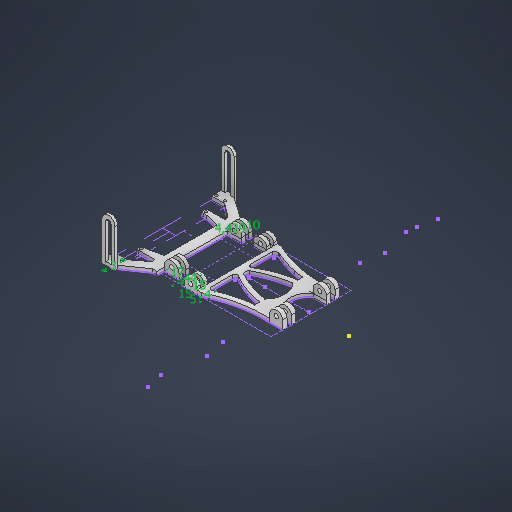
# Autodesk Inventor part: grebla2
Saved by Autodesk Inventor 2026.2 (Build 302298000, 298)
## iProperties
Created: 2026-03-31
Part Number: grebla2
Material: Generic
Document SubType Name: Modeling
Designer: Iosif
Density: 1 g/cm^3
Appearance: Default
Author: Iosif
Autodesk Inventor part; units mm, degrees
ref_plane "YZ Plane" through (0, 0, 0) normal (1, 0, 0) x (0, 1, 0)
ref_plane "XZ Plane" through (0, 0, 0) normal (0, 1, 0) x (-1, 0, 0)
ref_plane "XY Plane" through (0, 0, 0) normal (0, 0, 1) x (1, 0, 0)
sketch "Sketch1" plane through (0, 0, 0) normal (0, 1, 0) x (-1, 0, 0)
  line L0 (197.8218, 40) -> (201.8218, 40)
  arc A0 (201.8218, 34) -> (201.8218, 40) centre (201.8218, 37) ccw
  line L1 (201.8218, 34) -> (197.8218, 34)
  line L2 (197.8218, -34) -> (201.8218, -34)
  arc A1 (201.8218, -40) -> (201.8218, -34) centre (201.8218, -37) ccw
  line L3 (201.8218, -40) -> (197.8218, -40)
  line L4 (214.3218, -64) -> (214.3218, -59)
  line L5 (214.3218, -59) -> (214.3218, -56)
  line L6 (214.3218, -56) -> (199.3218, -56)
  line L7 (199.3218, 56) -> (214.3218, 56)
  line L8 (214.3218, 56) -> (214.3218, 59)
  line L9 (214.3218, 59) -> (214.3218, 64)
  line L10 (197.8218, 34) -> (182.1137, 30.3299)
  line L11 (182.1137, 30.3299) -> (182.1137, -30.3299)
  line L12 (182.1137, -30.3299) -> (197.8218, -34)
  line L13 (199.3218, 56) -> (184.6899, 44.9596)
  arc A2 (184.6899, 44.9596) -> (183.5786, 40) centre (187.0547, 41.8254) ccw
  line L14 (183.5786, 40) -> (197.8218, 40)
  line L15 (197.8218, -40) -> (183.5786, -40)
  arc A3 (183.5786, -40) -> (184.6899, -44.9596) centre (187.0547, -41.8254) ccw
  line L16 (184.6899, -44.9596) -> (199.3218, -56)
  line L17 (170.1376, 0) -> (214.3218, 0)
  line L18 (214.3218, 0) -> (214.3218, -64)
  line L19 (214.3218, 0) -> (214.3218, 64)
  line L20 (206.8218, 0) -> (206.8218, 59)
  line L21 (206.8218, 59) -> (214.3218, 59)
  line L22 (206.8218, 57.5) -> (211.8218, 57.5)
  line L23 (211.8218, 57.5) -> (211.8218, 59)
  line L24 (206.8218, 57.5) -> (201.8218, 57.5)
  line L25 (201.8218, 57.5) -> (201.8218, 59)
  circle A4 centre (211.8218, 59) radius 1.5
  circle A5 centre (201.8218, 59) radius 1.5
  circle A6 centre (211.8218, -59) radius 1.5
  circle A7 centre (201.8218, -59) radius 1.5
  line L26 (214.3218, 0) -> (214.3218, -64)
  line L27 (201.8218, 59) -> (201.8218, 37)
  circle A8 centre (201.8218, 37) radius 1.5
  circle A9 centre (201.8218, -37) radius 1.5
  line L28 (198.6427, 55.4876) -> (198.6427, 40)
  line L29 (198.6427, -56) -> (198.6427, -55.4876)
  line L30 (198.6427, -34.1918) -> (198.6427, -34)
  line L31 (199.3218, -8.7299) -> (189.3218, -8.7299)
  line L32 (199.3218, -56) -> (199.3218, -40)
  line L33 (199.3218, -34) -> (199.3218, 0)
  line L34 (199.3218, 56) -> (199.3218, 40)
  line L35 (199.3218, 34) -> (199.3218, 0)
  line L36 (183.5786, -40) -> (175.5622, -40)
  line L37 (214.3218, 64) -> (214.3218, 67)
  line L38 (214.3218, 67) -> (199.3218, 67)
  line L39 (199.3218, 67) -> (175.5622, 50.4798)
  line L40 (214.3218, -64) -> (214.3218, -67)
  line L41 (214.3218, -67) -> (199.3218, -67)
  line L42 (199.3218, -67) -> (175.5622, -50.4798)
  line L43 (175.5622, -50.4798) -> (170.5622, -50.4798)
  line L44 (170.5622, -50.4798) -> (170.5622, 50.4798)
  line L45 (170.5622, 50.4798) -> (175.5622, 50.4798)
  line L46 (63.8973, 32.5211) -> (58.8577, 32.5211)
  line L47 (58.8577, 32.5211) -> (58.8577, 17.5211)
  line L48 (58.8577, 17.5211) -> (58.8577, 32.5211)
  line L49 (58.8577, 32.5211) -> (58.8577, 17.5211)
  arc A10 (118.0743, 3.3266) -> (58.8577, 17.5211) centre (61.3775, -102.5839) ccw
  line L50 (58.8577, -17.4789) -> (58.8577, -32.3558)
  line L51 (58.8577, -32.3558) -> (63.8973, -32.3558)
  line L52 (63.8973, -27.1337) -> (63.8973, -27.0727)
  line L53 (63.8973, -17.4789) -> (58.8577, -17.4789)
  arc A11 (119.5352, 7.8267) -> (123.8577, 10.7806) centre (120.6872, 10.7806) ccw
  arc A12 (118.0743, -3.2843) -> (118.0549, 3.337) centre (115.0731, 0.0176) ccw
  line L54 (116.1179, 4.3839) -> (116.1009, 4.3596)
  line L55 (76.7429, 27.2559) -> (76.7429, 22.2861)
  line L56 (80.9342, 21.7713) -> (80.9342, 27.5805)
  line L57 (76.7429, -22.2438) -> (76.7429, -27.2136)
  line L58 (80.9342, -27.5382) -> (80.9342, -21.729)
  arc A13 (123.8577, 35.8089) -> (119.5352, 37.9363) centre (120.344, 34.1247) ccw
  arc A14 (119.5352, -37.894) -> (123.8577, -35.7666) centre (120.344, -34.0824) ccw
  line L59 (119.5352, -37.894) -> (117.8548, -37.894)
  arc A15 (123.8577, -10.7383) -> (119.5352, -7.7844) centre (120.6872, -10.7383) ccw
  line L60 (116.1179, 4.3839) -> (116.0752, 4.3728)
  line L61 (123.8577, 35.8089) -> (123.8577, 25.0211)
  line L62 (123.8577, 46.0935) -> (43.8577, 46.0935)
  line L63 (123.8577, -46.0512) -> (43.8577, -46.0512)
  line L64 (43.8577, -46.0512) -> (43.8577, 46.0935)
  line L65 (123.8577, 0.0211) -> (43.8577, 0.0211)
  line L66 (58.8577, 22.5211) -> (43.8577, 22.5211)
  line L67 (58.8577, 22.5211) -> (43.8577, 22.5211)
  line L68 (58.8577, 27.5211) -> (43.8577, 27.5211)
  line L69 (58.8577, 32.5211) -> (43.8577, 32.5211)
  line L70 (58.8577, 17.5211) -> (43.8577, 17.5211)
  arc A16 (58.8577, 32.5211) -> (123.8577, 46.0935) centre (64.6648, 167.1438) ccw
  line L71 (58.8577, -27.4789) -> (43.8577, -27.4789)
  line L72 (58.8577, -22.4789) -> (43.8577, -22.4789)
  line L73 (58.8577, -17.4789) -> (43.8577, -17.4789)
  line L74 (58.8577, -32.4789) -> (58.8577, -17.4789)
  line L75 (123.8577, 0.0211) -> (123.8577, 0)
  arc A17 (58.8577, -17.4789) -> (118.0743, -3.2843) centre (61.3775, 102.6262) ccw
  arc A18 (123.8577, -46.0512) -> (58.8577, -32.4789) centre (64.6648, -167.1015) ccw
  line L76 (123.8577, -46.0512) -> (43.8577, -46.0512)
  line L77 (123.8577, -35.7666) -> (123.8577, -24.9789)
  line L78 (58.8577, -32.4789) -> (43.8577, -32.4789)
  line L79 (63.8973, 17.5211) -> (58.8577, 17.5211)
  line L80 (58.8577, 17.5211) -> (58.8577, 32.5211)
  line L81 (63.8973, -32.3558) -> (58.8577, -32.3558)
  line L82 (58.8577, -32.3558) -> (58.8577, -17.4789)
  line L83 (123.8577, -22.4789) -> (170.5622, -22.4789) construction
  line L84 (123.8577, 22.5211) -> (170.5622, 22.5211) construction
  line L85 (123.8577, 46.0935) -> (170.5622, 46.0935) construction
  line L86 (123.8577, -46.0512) -> (170.5622, -46.0512) construction
  line L87 (170.5622, -46.0512) -> (160.5622, -46.0512) construction
  line L88 (160.5622, -46.0512) -> (160.5622, -49.9671) construction
  line L89 (123.8577, -46.0512) -> (149.8673, -46.0512) construction
  line L90 (149.8673, -46.0512) -> (149.8673, 46.0935) construction
  line L91 (123.8577, 46.0935) -> (128.8577, 46.0935)
  line L92 (128.8577, 46.0935) -> (128.8577, -46.0512)
  line L93 (123.8577, -46.0512) -> (128.8577, -46.0512)
  line L94 (128.8577, 46.0935) -> (143.8577, 46.0935)
  line L95 (143.8577, 46.0935) -> (143.8577, 42.0935)
  line L96 (143.8577, 42.0935) -> (128.8577, 42.0935)
  line L97 (128.8577, 42.0935) -> (128.8577, 38.0935)
  line L98 (128.8577, 38.0935) -> (143.8577, 38.0935)
  line L99 (143.8577, 38.0935) -> (143.8577, 34.0935)
  line L100 (143.8577, 34.0935) -> (128.8577, 34.0935)
  line L101 (170.5622, 42.0935) -> (143.8577, 42.0935) construction
  line L102 (143.8577, 38.0935) -> (170.5622, 38.0935) construction
  line L103 (170.5622, 42.0935) -> (153.5622, 42.0935)
  line L104 (153.5622, 42.0935) -> (153.5622, 38.0935)
  line L105 (170.5622, 38.0935) -> (153.5622, 38.0935)
  line L106 (170.5622, 34.0935) -> (153.5622, 34.0935)
  line L107 (153.5622, 34.0935) -> (153.5622, 30.0935)
  line L108 (153.5622, 30.0935) -> (170.5622, 30.0935)
  line L109 (128.8577, -46.0512) -> (143.8577, -46.0512)
  line L110 (143.8577, -46.0512) -> (143.8577, -42.0512)
  line L111 (143.8577, -42.0512) -> (128.8577, -42.0512)
  line L112 (128.8577, -38.0512) -> (143.8577, -38.0512)
  line L113 (143.8577, -38.0512) -> (143.8577, -34.0512)
  line L114 (143.8577, -34.0512) -> (128.8577, -34.0512)
  line L115 (170.5622, -42.0512) -> (153.5622, -42.0512)
  line L116 (153.5622, -42.0512) -> (153.5622, -38.0512)
  line L117 (170.5622, -38.0512) -> (153.5622, -38.0512)
  line L118 (170.5622, -34.0512) -> (153.5622, -34.0512)
  line L119 (153.5622, -34.0512) -> (153.5622, -30.0512)
  line L120 (153.5622, -30.0512) -> (170.5622, -30.0512)
  arc A19 (58.8577, -22.4789) -> (76.7429, -22.2438) centre (66.4719, 78.7041) ccw
  arc A20 (80.9342, -21.729) -> (119.5352, -7.7844) centre (66.4719, 78.7041) ccw
  arc A21 (58.8577, 27.5211) -> (76.7429, 27.2559) centre (69.5749, 147.0419) ccw
  arc A22 (80.9342, 27.5805) -> (119.5352, 37.9363) centre (69.5749, 147.0419) ccw
  arc A23 (119.5352, 7.8267) -> (80.9342, 21.7713) centre (66.4719, -78.6618) ccw
  arc A24 (76.7429, 22.2861) -> (58.8577, 22.5211) centre (66.4719, -78.6618) ccw
  arc A25 (119.5352, 7.8267) -> (80.9342, 21.7713) centre (66.4719, -78.6618) ccw
  arc A26 (76.7429, 22.2861) -> (58.8577, 22.5211) centre (66.4719, -78.6618) ccw
  arc A27 (58.8577, 27.5211) -> (76.7429, 27.2559) centre (69.5749, 147.0419) ccw
  arc A28 (80.9342, 27.5805) -> (119.5352, 37.9363) centre (69.5749, 147.0419) ccw
  line L121 (63.8973, 22.5211) -> (63.8973, 22.7746)
  line L122 (63.8973, 32.3981) -> (63.8973, 32.5211)
  arc A29 (58.8577, -22.4789) -> (76.7429, -22.2438) centre (66.4719, 78.7041) ccw
  arc A30 (80.9342, -21.729) -> (119.5352, -7.7844) centre (66.4719, 78.7041) ccw
  arc A31 (117.8548, -37.894) -> (80.9342, -27.4307) centre (70.1327, -135.9147) ccw
  arc A32 (76.7429, -27.0948) -> (58.8577, -27.4789) centre (70.1327, -135.9147) ccw
  arc A33 (119.5352, -37.894) -> (80.9342, -27.5382) centre (69.5749, -146.9996) ccw
  arc A34 (63.8973, -27.1337) -> (58.8577, -27.4789) centre (69.5749, -146.9996) ccw
  line L123 (74.4899, -22.4789) -> (74.0861, -22.4789)
  line L124 (58.8577, -22.4789) -> (43.8577, -22.4789)
  arc A35 (118.0549, -3.2947) -> (118.0743, 3.3266) centre (115.0731, 0.0247) ccw
  arc A36 (116.1052, 4.3658) -> (116.0752, 4.3728) centre (115.0731, 0.0247) ccw
  line L125 (123.8577, -39.9789) -> (123.8577, -40)
  line L126 (123.8577, 35.8089) -> (123.8577, 10.7806)
  line L127 (123.8577, -10.7383) -> (123.8577, -35.7666)
  line L128 (123.8577, -35.7666) -> (123.8577, -10.7383)
  line L129 (123.8577, 10.7806) -> (123.8577, 35.8089)
  arc A37 (58.8577, -17.4789) -> (58.8577, 17.5211) centre (46.1869, 0.0211) ccw
  arc A38 (80.9342, 15.945) -> (80.9342, -15.9027) centre (96.6874, 0.0211) ccw
  point P0 (0, 0)
  point P1 (183.5786, 40)
  point P2 (123.8577, 46.0935)
  point P3 (118.0743, 3.3266)
  point P4 (92.2366, -29.1586)
  dimension "d0" = 3
  dimension "d11" = 4.4286
  dimension "d12" = 10
  dimension "d14" = 5
  dimension "d15" = 15
  dimension "d16" = 4
  dimension "d17" = 15
  dimension "d18" = 4
  dimension "d19" = 4
  dimension "d20" = 17
  dimension "d21" = 4
  constraints: 258 end point, 74 point on circle, 39 centre point, 25 point on line, 19 symmetric about line, 9 horizontal, 9 perpendicular, 1 collinear, 1 parallel, 1 vertical, 11 other
  measures "d0" distance of L37.start L37.end
  measures "d11" distance of L86.end L43.end
  measures "d12" distance of L86.end L87.end
  measures "d14" distance of L85.start L91.end
  measures "d15" distance of L91.end L94.end
  measures "d16" distance of L94.end L95.end
  measures "d17" distance of L95.end L96.end
  measures "d18" distance of L96.end L97.end
  measures "d19" distance of L98.end L99.end
  measures "d20" distance of L101.start L103.end
  measures "d21" distance of L106.end L107.end
extrude "Extrusion1" add sketch "Sketch1" along normal blind 4 contours L0 A0 L1 L10 L11 L17 L44 L45 L39 L38 L37 L9 L21 A4 L20 L24 L27 L7 L13 A2 L14 | L27 L24 L20 L7 | L20 L22 A4 L21 L8 L7 | L20 L21 A4 L22 | L11 L12 L2 A1 L3 L15 A3 L16 L6 L5 L4 L40 L41 L42 L43 L44 L17 | L44 L118 L119 L120 | L108 L107 L106 L44 | L44 L115 L116 L117 | L105 L104 L103 L44 | A16 L91 L92 L93 A18 L51 L50 A34 L52 A32 L57 A19 A17 A12 A35 A10 L54 L60 L47 A24 L55 A21 | L47 L68 L64 L69 | A21 L55 A24 L47 | L47 L70 L64 L66 | L94 L95 L96 L92 | L79 A10 A38 L65 A37 | L65 A38 A17 L53 A37 | L98 L99 L100 L92 | L50 L72 L64 L73 | A19 L57 A32 L50 | L114 L113 L112 L92 | L50 L74 L78 L64 L71 | A32 L52 A34 | L111 L110 L109 L92
sketch "Sketch2" plane through (-214.3218, 0, 67) normal (0, 0, 1) x (1, 0, 0)
  line L0 (0, 0) -> (0, 4) projected
  line L1 (0, 0) -> (0, 4)
  line L2 (0, 4) -> (0, 44)
  line L3 (15, 0) -> (15, 4) projected
  line L4 (15, 4) -> (15, 44)
  arc A0 (15, 44) -> (0, 44) centre (7.5, 44) ccw
  arc A1 (10.5, 44) -> (4.5, 44) centre (7.5, 44) ccw
  line L5 (4.5, 44) -> (4.5, 4)
  line L6 (4.5, 4) -> (10.5, 4)
  line L7 (10.5, 4) -> (10.5, 44)
  line L8 (0, 0) -> (15, 0) projected
  line L9 (0, 0) -> (15, 0)
  line L10 (0, 4) -> (15, 4) projected
  line L11 (15, 4) -> (38.7595, 4) projected
  line L12 (38.7595, 4) -> (43.7595, 4) projected
  line L13 (43.7595, 4) -> (38.7595, 4) projected
  line L14 (38.7595, 4) -> (15, 4) projected
  line L15 (15, 4) -> (0, 4) projected
  line L16 (0, 4) -> (15, 4) projected
  line L17 (15, 4) -> (29.6319, 4) projected
  line L18 (29.6319, 4) -> (30.7431, 4) projected
  line L19 (30.7431, 4) -> (12.5, 4) projected
  line L20 (12.5, 4) -> (12.5, 4) projected
  line L21 (12.5, 4) -> (16.5, 4) projected
  line L22 (16.5, 4) -> (32.2081, 4) projected
  line L23 (32.2081, 4) -> (16.5, 4) projected
  line L24 (16.5, 4) -> (12.5, 4) projected
  line L25 (12.5, 4) -> (12.5, 4) projected
  line L26 (12.5, 4) -> (30.7431, 4) projected
  line L27 (30.7431, 4) -> (29.6319, 4) projected
  line L28 (29.6319, 4) -> (15, 4) projected
  line L29 (15, 4) -> (0, 4) projected
  line L30 (1, 4) -> (4, 4) projected
  line L31 (11, 4) -> (14, 4) projected
  line L32 (11, 4) -> (14, 4) projected
  line L33 (1, 4) -> (4, 4) projected
  line L34 (11, 4) -> (14, 4) projected
  line L35 (11, 4) -> (14, 4) projected
  line L36 (43.7595, 4) -> (60.7595, 4) projected
  line L37 (60.7595, 4) -> (43.7595, 4) projected
  line L38 (43.7595, 4) -> (60.7595, 4) projected
  line L39 (60.7595, 4) -> (43.7595, 4) projected
  line L40 (43.7595, 4) -> (60.7595, 4) projected
  line L41 (60.7595, 4) -> (43.7595, 4) projected
  line L42 (43.7595, 4) -> (60.7595, 4) projected
  line L43 (60.7595, 4) -> (43.7595, 4) projected
  point P0 (214.3218, 0)
  dimension "d4" = 6
  constraints: 14 end point, 4 point on circle, 2 centre point, 2 collinear, 2 tangent, 2 vertical, 1 coincident, 1 perpendicular, 1 point on line
  measures "d4" diameter of A1
extrude "Extrusion2" add sketch "Sketch2" along normal blind 3 contours L0 L10 L6 L3 L8 | L2 A0 L4 L10 L7 A1 L5
sketch "Sketch3" plane through (-199.3218, 0, -67) normal (0, 0, -1) x (-1, 0, 0)
  line L0 (-15.7431, 0) -> (2.5, 0) projected
  line L1 (0, 4) -> (0, 44) projected
  line L2 (0, 0) -> (0, 44)
  line L3 (0, 0) -> (15, 0)
  arc A0 (15, 44) -> (0, 44) centre (7.5, 44) ccw projected
  arc A1 (15, 44) -> (0, 44) centre (7.5, 44) ccw
  line L4 (0, 4) -> (15, 4) projected
  line L5 (4.5, 4) -> (10.5362, 4)
  line L6 (10.5, 4) -> (10.5, 44) projected
  line L7 (4.5, 44) -> (4.5, 4) projected
  line L8 (4.5, 4) -> (4.5, 44)
  arc A2 (10.5, 44) -> (4.5, 44) centre (7.5, 44) ccw
  line L9 (15, 44) -> (15, 0)
  point P0 (-199.3218, 0)
  constraints: 10 end point, 4 point on circle, 3 point on line, 3 tangent, 2 centre point, 2 collinear, 1 horizontal, 1 vertical
extrude "Extrusion3" add sketch "Sketch3" along normal blind 3 contours L2 L4 L9 L3 L0 | L1 A0 L9 L4 L6 A2 L7
sketch "Sketch4" plane through (-170.5622, 0, 42.0935) normal (0, 0, 1) x (1, 0, 0)
  line L0 (0, 0) -> (17, 0) projected
  line L1 (8.5, 0) -> (8.5, 8)
  circle A0 centre (8.5, 8) radius 2.5
  line L2 (-5, 0) -> (0, 0) projected
  line L3 (0, 0) -> (0, 6)
  line L4 (17, 0) -> (17, 6)
  arc A1 (17, 6) -> (0, 6) centre (8.5, 6) ccw
  line L5 (0, 4) -> (-5, 4) projected
  line L6 (0, 4) -> (0, 0)
  line L7 (0, 4) -> (17, 4)
  point P0 (170.5622, 0)
  dimension "d22" = 8
  dimension "d23" = 5
  dimension "d24" = 6
  constraints: 10 end point, 3 vertical, 2 centre point, 2 point on circle, 2 tangent, 1 coincident, 1 collinear, 1 midpoint, 1 perpendicular, 1 point on line
  measures "d22" distance of L1.start L1.end
  measures "d23" diameter of A0
  measures "d24" distance of L0.start L3.end
extrude "Extrusion4" add sketch "Sketch4" against normal blind 4 contours L3 A1 L4 L7
sketch "Sketch5" plane through (-153.5622, 0, 30.0935) normal (0, 0, -1) x (-1, 0, 0)
  circle A0 centre (8.5, 8) radius 2.5 projected
  circle A1 centre (8.5, 8) radius 2.5
  arc A2 (17, 6) -> (0, 6) centre (8.5, 6) ccw projected
  arc A3 (17, 6) -> (0, 6) centre (8.5, 6) ccw
  line L0 (0, 0) -> (0, 6) projected
  line L1 (17, 4) -> (0, 4) projected
  line L2 (0, 6) -> (0, 4)
  line L3 (0, 4) -> (17, 4)
  line L4 (17, 4) -> (17, 6)
  point P0 (-153.5622, 0)
  constraints: 6 end point, 2 centre point, 2 point on circle, 1 coincident, 1 collinear, 1 perpendicular, 1 vertical
extrude "Extrusion5" add sketch "Sketch5" against normal blind 4
mirror "Mirror2" about plane through (0, 0, 0) normal (0, 0, 1) of "Extrusion4", "Extrusion5"
sketch "Sketch6" plane through (-143.8577, 0, 46.0935) normal (0, 0, 1) x (1, 0, 0)
  line L0 (-11.7045, 4) -> (-11.7045, 4.1096)
  circle A0 centre (7.5438, 6.5964) radius 2.5
  circle A1 centre (7.5438, 6.5964) radius 2.5
  line L1 (0, 6.1096) -> (0, 4.1096)
  line L2 (0, 6.1096) -> (0, 4.1096)
  line L3 (15, 4.1096) -> (15, 6.1096)
  line L4 (0, 4.1096) -> (0, 4)
  line L5 (0, 0) -> (0, 4) projected
  line L6 (15, 4) -> (15, 4.1096)
  line L7 (-11.9432, 4) -> (-11.7045, 4)
  arc A2 (15, 7.3498) -> (0, 7.4214) centre (7.4855, 4.3452) ccw
  line L8 (0, 7.4214) -> (0, 6.1096)
  line L9 (15, 7.3498) -> (15, 6.1096)
  line L10 (15, 4.1096) -> (15, 4)
  line L11 (0, 4) -> (15, 4)
  point P0 (143.8577, 0)
  point P1 (0, 3.2406)
  dimension "d31" = 15
  constraints: 22 end point, 4 point on line, 3 centre point, 2 collinear, 2 parallel, 2 point on circle, 1 coincident, 1 horizontal, 1 perpendicular, 1 vertical
  measures "d31" distance of L3.start L1.end
extrude "Extrusion6" add sketch "Sketch6" against normal blind 4
sketch "Sketch7" plane through (-128.8577, 0, 34.0935) normal (0, 0, -1) x (-1, 0, 0)
  circle A0 centre (7.4562, 6.5964) radius 2.5 projected
  circle A1 centre (7.4562, 6.5964) radius 2.5
  arc A2 (15, 7.4214) -> (0, 7.3498) centre (7.5145, 4.3452) ccw
  line L0 (0, 7.3498) -> (0, 4)
  line L1 (15, 3.7107) -> (15, 7.4214)
  line L2 (15, 7.4214) -> (15, 4)
  line L3 (15, 4) -> (0, 4)
  point P0 (-128.8577, 0)
  constraints: 8 end point, 2 centre point, 2 point on circle, 1 coincident, 1 collinear
extrude "Extrusion7" add sketch "Sketch7" against normal blind 4
mirror "Mirror3" about plane through (0, 0, 0) normal (0, 0, 1) of "Extrusion7", "Extrusion6"
sketch "Sketch8" plane through (-58.8577, 0, 32.5211) normal (0, 0, 1) x (1, 0, 0)
  line L0 (0, 0) -> (0, 4) construction
  line L1 (0, 0) -> (15, 0) construction
  line L2 (0, 0) -> (15, 0) construction
  line L3 (15, 0) -> (7.5, 0) construction
  line L4 (7.5, 10) -> (7.5, 0) construction
  line L5 (0, 4) -> (15, 4) construction
  circle A0 centre (7.5, 10) radius 2.5
  arc A1 (15, 10) -> (0, 10) centre (7.5, 8.5149) ccw
  line L6 (0, 10) -> (0, 4)
  line L7 (15, 4) -> (15, 10)
  line L8 (0, 4) -> (15, 4)
  point P0 (58.8577, 0)
  dimension "d34" = 5
  dimension "d35" = 10
  constraints: 12 end point, 3 equal length, 2 centre point, 2 midpoint, 2 point on circle, 1 coincident, 1 perpendicular, 1 vertical
  measures "d34" diameter of A0
  measures "d35" distance of point (7.5, 0) L4.start
extrude "Extrusion8" add sketch "Sketch8" against normal blind 5
sketch "Sketch9" plane through (-43.8577, 0, 17.5211) normal (0, 0, -1) x (-1, 0, 0)
  circle A0 centre (7.5, 10) radius 2.5 projected
  circle A1 centre (7.5, 10) radius 2.5
  line L0 (15, 4) -> (15, 10) projected
  line L1 (0, 0) -> (0, 10) projected
  arc A2 (15, 10) -> (0, 10) centre (7.5, 8.5149) ccw
  arc A3 (15, 10) -> (0, 10) centre (7.5, 8.5149) ccw projected
  line L2 (15, 4) -> (20.0396, 4) projected
  line L3 (0, 4) -> (15, 4)
  point P0 (-43.8577, 0)
  constraints: 2 centre point, 2 end point, 2 point on circle, 1 coincident, 1 collinear, 1 concentric, 1 point on line
extrude "Extrusion9" add sketch "Sketch9" against normal blind 5
mirror "Mirror4" about plane through (0, 0, 0) normal (0, 0, 1) of "Extrusion9", "Extrusion8"
body "Solid1"
